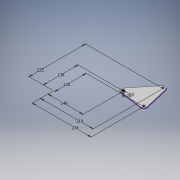
# Autodesk Inventor part: ternary_link
Saved by Autodesk Inventor 2019 (Build 230136000, 136)
## iProperties
Created: 2021-02-18
Part Number: ternary_link
Material: 一般
Document SubType Name: Modeling
Designer: wasd5
Density: 1 g/cm^3
Appearance: 預設
Author: wasd5
Autodesk Inventor part; units mm, degrees
ref_plane "YZ Plane" through (0, 0, 0) normal (1, 0, 0) x (0, 1, 0)
ref_plane "XZ Plane" through (0, 0, 0) normal (0, 1, 0) x (-1, 0, 0)
ref_plane "XY Plane" through (0, 0, 0) normal (0, 0, 1) x (1, 0, 0)
sketch "草圖2" plane through (0, 0, 0) normal (0, 1, 0) x (-1, 0, 0)
  line L0 (-234, -125) -> (-210, -225) construction
  line L1 (-210, -225) -> (-140, -138) construction
  arc A0 (-132.2088, -144.2688) -> (-138.6301, -128.0943) centre (-140, -138) ccw
  arc A1 (-219.7239, -227.3337) -> (-202.2088, -231.2688) centre (-210, -225) ccw
  line L2 (-132.2088, -144.2688) -> (-202.2088, -231.2688)
  line L3 (-138.6301, -128.0943) -> (-232.6301, -115.0943)
  line L4 (-140, -138) -> (-234, -125) construction
  arc A2 (-232.6301, -115.0943) -> (-243.7239, -127.3337) centre (-234, -125) ccw
  line L5 (-219.7239, -227.3337) -> (-243.7239, -127.3337)
  circle A3 centre (-140, -138) radius 5
  circle A4 centre (-210, -225) radius 5
  circle A5 centre (-234, -125) radius 5
  point P0 (0, 0)
  dimension "d11" = 20
  dimension "hole" = 10
  dimension "x1" = 140
  dimension "y1" = 138
  dimension "x3" = 234
  dimension "y3" = 125
  dimension "y2" = 225
  dimension "x2" = 210
  constraints: 12 end point, 6 centre point, 6 coincident, 6 point on circle, 6 tangent, 4 equal radius
  measures "d11" diameter of A0
  measures "hole" diameter of A3
  measures "x1" horizontal distance of point (0, 0) A3.centre
  measures "y1" vertical distance of A3.centre point (0, 0)
  measures "x3" horizontal distance of A5.centre point (0, 0)
  measures "y3" vertical distance of point (0, 0) A5.centre
  measures "y2" vertical distance of point (0, 0) A4.centre
  measures "x2" horizontal distance of point (0, 0) A4.centre
extrude "擠出2" add sketch "草圖2" along normal blind 3
equation "\"d11\" = 2 * hole"
